Autodesk Fusion 360 part; units mm, degrees
(part 6 of 7)
  spline S7 degree 5 poles (-3.0907, -4.5495) (-3.0883, -4.5484) (-3.0835, -4.5462) (-3.0762, -4.5428) (-3.0666, -4.5384) (-3.0547, -4.5328) (-3.0428, -4.5271) (-3.0309, -4.5214) (-3.0191, -4.5157) (-3.0074, -4.5099) (-2.9957, -4.504) (-2.984, -4.4981) (-2.9724, -4.4922) (-2.9609, -4.4862) (-2.9494, -4.4802) (-2.9379, -4.4741) (-2.9265, -4.468) (-2.9152, -4.4618) (-2.9039, -4.4556) (-2.8926, -4.4494) (-2.8814, -4.443) (-2.8703, -4.4367) (-2.8592, -4.4303) (-2.8482, -4.4238) (-2.8372, -4.4173) (-2.8263, -4.4108) (-2.8154, -4.4042) (-2.8046, -4.3976) (-2.7939, -4.3909) (-2.7832, -4.3841) (-2.7726, -4.3773) (-2.762, -4.3705) (-2.7515, -4.3636) (-2.741, -4.3567) (-2.7306, -4.3497) (-2.7203, -4.3427) (-2.71, -4.3356) (-2.6998, -4.3285) (-2.6897, -4.3213) (-2.6796, -4.3141) (-2.6696, -4.3068) (-2.6597, -4.2995) (-2.6498, -4.2921) (-2.64, -4.2847) (-2.6303, -4.2772) (-2.6206, -4.2697) (-2.611, -4.2621) (-2.6015, -4.2544) (-2.5921, -4.2467) (-2.5827, -4.239) (-2.5734, -4.2312) (-2.5642, -4.2233) (-2.5551, -4.2154) (-2.5461, -4.2074) (-2.5371, -4.1994) (-2.5282, -4.1913) (-2.5195, -4.1831) (-2.5107, -4.1749) (-2.5021, -4.1667) (-2.4936, -4.1583) (-2.4852, -4.1499) (-2.4769, -4.1415) (-2.4687, -4.1329) (-2.4607, -4.1242) (-2.4528, -4.1155) (-2.445, -4.1067) (-2.4373, -4.0978) (-2.4297, -4.0889) (-2.4221, -4.08) (-2.4148, -4.0709) (-2.4077, -4.0616) (-2.4024, -4.054) (-2.3986, -4.0482) (-2.3962, -4.0442) (-2.395, -4.0422) knots -1 -1 -1 -1 -1 -1 -0.98571429 -0.97142857 -0.95714286 -0.94285714 -0.92857143 -0.91428571 -0.9 -0.88571429 -0.87142857 -0.85714286 -0.84285714 -0.82857143 -0.81428571 -0.8 -0.78571429 -0.77142857 -0.75714286 -0.74285714 -0.72857143 -0.71428571 -0.7 -0.68571429 -0.67142857 -0.65714286 -0.64285714 -0.62857143 -0.61428571 -0.6 -0.58571429 -0.57142857 -0.55714286 -0.54285714 -0.52857143 -0.51428571 -0.5 -0.48571429 -0.47142857 -0.45714286 -0.44285714 -0.42857143 -0.41428571 -0.4 -0.38571429 -0.37142857 -0.35714286 -0.34285714 -0.32857143 -0.31428571 -0.3 -0.28571429 -0.27142857 -0.25714286 -0.24285714 -0.22857143 -0.21428571 -0.2 -0.18571429 -0.17142857 -0.15714286 -0.14285714 -0.12857143 -0.11428571 -0.1 -0.08571429 -0.07142857 -0.05714286 -0.04285714 -0.02857143 -0.01428571 0 0 0 0 0 0
  line L7 (-2.395, -4.0422) -> (-2.2666, -3.8269)
  arc A15 (-2.1317, -3.791) -> (-2.2666, -3.8269) centre (-2.1807, -3.8781) ccw
  arc A16 (-2.1317, -3.791) -> (-1.814, -3.9529) centre (0, 0) ccw
  arc A17 (-1.7637, -4.0832) -> (-1.814, -3.9529) centre (-1.8557, -4.0437) ccw
  line L8 (-1.7637, -4.0832) -> (-1.8625, -4.3135)
  spline S8 degree 5 poles (-1.8625, -4.3135) (-1.8634, -4.3157) (-1.8652, -4.32) (-1.8677, -4.3265) (-1.8707, -4.3353) (-1.8741, -4.3464) (-1.8771, -4.3577) (-1.8799, -4.3691) (-1.8826, -4.3805) (-1.8852, -4.3919) (-1.8877, -4.4034) (-1.8902, -4.4149) (-1.8925, -4.4265) (-1.8946, -4.4381) (-1.8966, -4.4498) (-1.8985, -4.4616) (-1.9002, -4.4734) (-1.9018, -4.4852) (-1.9033, -4.4971) (-1.9047, -4.509) (-1.9061, -4.5209) (-1.9073, -4.5329) (-1.9085, -4.5449) (-1.9095, -4.5569) (-1.9105, -4.569) (-1.9113, -4.5811) (-1.9121, -4.5932) (-1.9128, -4.6054) (-1.9134, -4.6176) (-1.9139, -4.6298) (-1.9143, -4.642) (-1.9146, -4.6543) (-1.9149, -4.6666) (-1.915, -4.6789) (-1.9151, -4.6913) (-1.9151, -4.7036) (-1.9151, -4.716) (-1.9149, -4.7284) (-1.9147, -4.7409) (-1.9144, -4.7533) (-1.914, -4.7658) (-1.9135, -4.7783) (-1.913, -4.7909) (-1.9124, -4.8034) (-1.9117, -4.816) (-1.9109, -4.8286) (-1.9101, -4.8412) (-1.9092, -4.8538) (-1.9082, -4.8664) (-1.9072, -4.8791) (-1.906, -4.8918) (-1.9048, -4.9045) (-1.9036, -4.9172) (-1.9022, -4.9299) (-1.9008, -4.9427) (-1.8994, -4.9554) (-1.8978, -4.9682) (-1.8962, -4.981) (-1.8945, -4.9938) (-1.8928, -5.0066) (-1.891, -5.0195) (-1.8891, -5.0323) (-1.8871, -5.0452) (-1.8851, -5.0581) (-1.883, -5.071) (-1.8809, -5.0839) (-1.8787, -5.0968) (-1.8764, -5.1097) (-1.874, -5.1227) (-1.8716, -5.1356) (-1.8691, -5.1486) (-1.8671, -5.1589) (-1.8655, -5.1667) (-1.8645, -5.1719) (-1.8639, -5.1745) knots 0 0 0 0 0 0 0.01428571 0.02857143 0.04285714 0.05714286 0.07142857 0.08571429 0.1 0.11428571 0.12857143 0.14285714 0.15714286 0.17142857 0.18571429 0.2 0.21428571 0.22857143 0.24285714 0.25714286 0.27142857 0.28571429 0.3 0.31428571 0.32857143 0.34285714 0.35714286 0.37142857 0.38571429 0.4 0.41428571 0.42857143 0.44285714 0.45714286 0.47142857 0.48571429 0.5 0.51428571 0.52857143 0.54285714 0.55714286 0.57142857 0.58571429 0.6 0.61428571 0.62857143 0.64285714 0.65714286 0.67142857 0.68571429 0.7 0.71428571 0.72857143 0.74285714 0.75714286 0.77142857 0.78571429 0.8 0.81428571 0.82857143 0.84285714 0.85714286 0.87142857 0.88571429 0.9 0.91428571 0.92857143 0.94285714 0.95714286 0.97142857 0.98571429 1 1 1 1 1 1
  arc A18 (-1.8639, -5.1745) -> (-1.5336, -5.2819) centre (0, 0) ccw
  spline S9 degree 5 poles (-1.5336, -5.2819) (-1.5316, -5.2801) (-1.5277, -5.2765) (-1.5219, -5.2711) (-1.5141, -5.2639) (-1.5045, -5.2549) (-1.4949, -5.2458) (-1.4854, -5.2367) (-1.476, -5.2276) (-1.4666, -5.2185) (-1.4572, -5.2093) (-1.448, -5.2001) (-1.4388, -5.1909) (-1.4296, -5.1816) (-1.4206, -5.1723) (-1.4115, -5.163) (-1.4026, -5.1537) (-1.3937, -5.1443) (-1.3849, -5.1349) (-1.3761, -5.1255) (-1.3674, -5.116) (-1.3588, -5.1065) (-1.3502, -5.097) (-1.3417, -5.0875) (-1.3333, -5.0779) (-1.3249, -5.0683) (-1.3167, -5.0587) (-1.3084, -5.049) (-1.3003, -5.0393) (-1.2922, -5.0296) (-1.2842, -5.0199) (-1.2762, -5.0101) (-1.2684, -5.0003) (-1.2606, -4.9905) (-1.2528, -4.9806) (-1.2452, -4.9708) (-1.2376, -4.9609) (-1.2301, -4.9509) (-1.2227, -4.941) (-1.2154, -4.931) (-1.2081, -4.921) (-1.2009, -4.9109) (-1.1938, -4.9009) (-1.1868, -4.8908) (-1.1798, -4.8807) (-1.173, -4.8705) (-1.1662, -4.8603) (-1.1595, -4.8501) (-1.1529, -4.8399) (-1.1464, -4.8296) (-1.14, -4.8193) (-1.1336, -4.809) (-1.1274, -4.7987) (-1.1213, -4.7883) (-1.1153, -4.7779) (-1.1093, -4.7674) (-1.1035, -4.7569) (-1.0977, -4.7465) (-1.0921, -4.7359) (-1.0865, -4.7254) (-1.0811, -4.7148) (-1.0759, -4.7042) (-1.0708, -4.6935) (-1.0659, -4.6828) (-1.061, -4.672) (-1.0564, -4.6612) (-1.0517, -4.6504) (-1.0472, -4.6396) (-1.0428, -4.6288) (-1.0386, -4.6179) (-1.0348, -4.6069) (-1.032, -4.598) (-1.0302, -4.5913) (-1.0291, -4.5868) (-1.0286, -4.5845) knots -1 -1 -1 -1 -1 -1 -0.98571429 -0.97142857 -0.95714286 -0.94285714 -0.92857143 -0.91428571 -0.9 -0.88571429 -0.87142857 -0.85714286 -0.84285714 -0.82857143 -0.81428571 -0.8 -0.78571429 -0.77142857 -0.75714286 -0.74285714 -0.72857143 -0.71428571 -0.7 -0.68571429 -0.67142857 -0.65714286 -0.64285714 -0.62857143 -0.61428571 -0.6 -0.58571429 -0.57142857 -0.55714286 -0.54285714 -0.52857143 -0.51428571 -0.5 -0.48571429 -0.47142857 -0.45714286 -0.44285714 -0.42857143 -0.41428571 -0.4 -0.38571429 -0.37142857 -0.35714286 -0.34285714 -0.32857143 -0.31428571 -0.3 -0.28571429 -0.27142857 -0.25714286 -0.24285714 -0.22857143 -0.21428571 -0.2 -0.18571429 -0.17142857 -0.15714286 -0.14285714 -0.12857143 -0.11428571 -0.1 -0.08571429 -0.07142857 -0.05714286 -0.04285714 -0.02857143 -0.01428571 0 0 0 0 0 0
  line L9 (-1.0286, -4.5845) -> (-0.9731, -4.34)
  arc A19 (-0.8559, -4.2641) -> (-0.9731, -4.34) centre (-0.8756, -4.3622) ccw
  arc A20 (-0.8559, -4.2641) -> (-0.5037, -4.3199) centre (0, 0) ccw
  arc A21 (-0.4157, -4.4283) -> (-0.5037, -4.3199) centre (-0.5152, -4.4193) ccw
  line L10 (-0.4157, -4.4283) -> (-0.4384, -4.678)
  spline S10 degree 5 poles (-0.4384, -4.678) (-0.4386, -4.6803) (-0.439, -4.6849) (-0.4393, -4.6919) (-0.4395, -4.7012) (-0.4392, -4.7128) (-0.4386, -4.7245) (-0.4378, -4.7361) (-0.4368, -4.7478) (-0.4357, -4.7595) (-0.4346, -4.7712) (-0.4334, -4.7829) (-0.432, -4.7947) (-0.4304, -4.8064) (-0.4287, -4.8181) (-0.4269, -4.8299) (-0.4248, -4.8416) (-0.4227, -4.8534) (-0.4205, -4.8651) (-0.4182, -4.8769) (-0.4158, -4.8886) (-0.4133, -4.9004) (-0.4106, -4.9122) (-0.4079, -4.9239) (-0.4051, -4.9357) (-0.4022, -4.9475) (-0.3991, -4.9593) (-0.396, -4.971) (-0.3928, -4.9828) (-0.3895, -4.9946) (-0.3861, -5.0064) (-0.3826, -5.0181) (-0.3791, -5.0299) (-0.3754, -5.0417) (-0.3717, -5.0535) (-0.3679, -5.0652) (-0.364, -5.077) (-0.36, -5.0888) (-0.3559, -5.1005) (-0.3518, -5.1123) (-0.3476, -5.124) (-0.3433, -5.1358) (-0.3389, -5.1475) (-0.3344, -5.1593) (-0.3299, -5.171) (-0.3253, -5.1828) (-0.3206, -5.1945) (-0.3158, -5.2062) (-0.311, -5.2179) (-0.3061, -5.2297) (-0.3011, -5.2414) (-0.296, -5.2531) (-0.2909, -5.2648) (-0.2857, -5.2765) (-0.2804, -5.2882) (-0.2751, -5.2998) (-0.2697, -5.3115) (-0.2642, -5.3232) (-0.2586, -5.3348) (-0.253, -5.3465) (-0.2473, -5.3581) (-0.2415, -5.3698) (-0.2357, -5.3814) (-0.2298, -5.393) (-0.2238, -5.4047) (-0.2178, -5.4163) (-0.2117, -5.4279) (-0.2055, -5.4395) (-0.1993, -5.451) (-0.193, -5.4626) (-0.1866, -5.4742) (-0.1815, -5.4834) (-0.1776, -5.4903) (-0.175, -5.4949) (-0.1737, -5.4973) knots 0 0 0 0 0 0 0.01428571 0.02857143 0.04285714 0.05714286 0.07142857 0.08571429 0.1 0.11428571 0.12857143 0.14285714 0.15714286 0.17142857 0.18571429 0.2 0.21428571 0.22857143 0.24285714 0.25714286 0.27142857 0.28571429 0.3 0.31428571 0.32857143 0.34285714 0.35714286 0.37142857 0.38571429 0.4 0.41428571 0.42857143 0.44285714 0.45714286 0.47142857 0.48571429 0.5 0.51428571 0.52857143 0.54285714 0.55714286 0.57142857 0.58571429 0.6 0.61428571 0.62857143 0.64285714 0.65714286 0.67142857 0.68571429 0.7 0.71428571 0.72857143 0.74285714 0.75714286 0.77142857 0.78571429 0.8 0.81428571 0.82857143 0.84285714 0.85714286 0.87142857 0.88571429 0.9 0.91428571 0.92857143 0.94285714 0.95714286 0.97142857 0.98571429 1 1 1 1 1 1
  arc A22 (-0.1737, -5.4973) -> (0.1737, -5.4973) centre (0, 0) ccw
  spline S11 degree 5 poles (0.1737, -5.4973) (0.175, -5.4949) (0.1776, -5.4903) (0.1815, -5.4834) (0.1866, -5.4742) (0.193, -5.4626) (0.1993, -5.451) (0.2055, -5.4395) (0.2117, -5.4279) (0.2178, -5.4163) (0.2238, -5.4047) (0.2298, -5.393) (0.2357, -5.3814) (0.2415, -5.3698) (0.2473, -5.3581) (0.253, -5.3465) (0.2586, -5.3348) (0.2642, -5.3232) (0.2697, -5.3115) (0.2751, -5.2998) (0.2804, -5.2882) (0.2857, -5.2765) (0.2909, -5.2648) (0.296, -5.2531) (0.3011, -5.2414) (0.3061, -5.2297) (0.311, -5.2179) (0.3158, -5.2062) (0.3206, -5.1945) (0.3253, -5.1828) (0.3299, -5.171) (0.3344, -5.1593) (0.3389, -5.1475) (0.3433, -5.1358) (0.3476, -5.124) (0.3518, -5.1123) (0.3559, -5.1005) (0.36, -5.0888) (0.364, -5.077) (0.3679, -5.0652) (0.3717, -5.0535) (0.3754, -5.0417) (0.3791, -5.0299) (0.3826, -5.0181) (0.3861, -5.0064) (0.3895, -4.9946) (0.3928, -4.9828) (0.396, -4.971) (0.3991, -4.9593) (0.4022, -4.9475) (0.4051, -4.9357) (0.4079, -4.9239) (0.4106, -4.9122) (0.4133, -4.9004) (0.4158, -4.8886) (0.4182, -4.8769) (0.4205, -4.8651) (0.4227, -4.8534) (0.4248, -4.8416) (0.4269, -4.8299) (0.4287, -4.8181) (0.4304, -4.8064) (0.432, -4.7947) (0.4334, -4.7829) (0.4346, -4.7712) (0.4357, -4.7595) (0.4368, -4.7478) (0.4378, -4.7361) (0.4386, -4.7245) (0.4392, -4.7128) (0.4395, -4.7012) (0.4393, -4.6919) (0.439, -4.6849) (0.4386, -4.6803) (0.4384, -4.678) knots -1 -1 -1 -1 -1 -1 -0.98571429 -0.97142857 -0.95714286 -0.94285714 -0.92857143 -0.91428571 -0.9 -0.88571429 -0.87142857 -0.85714286 -0.84285714 -0.82857143 -0.81428571 -0.8 -0.78571429 -0.77142857 -0.75714286 -0.74285714 -0.72857143 -0.71428571 -0.7 -0.68571429 -0.67142857 -0.65714286 -0.64285714 -0.62857143 -0.61428571 -0.6 -0.58571429 -0.57142857 -0.55714286 -0.54285714 -0.52857143 -0.51428571 -0.5 -0.48571429 -0.47142857 -0.45714286 -0.44285714 -0.42857143 -0.41428571 -0.4 -0.38571429 -0.37142857 -0.35714286 -0.34285714 -0.32857143 -0.31428571 -0.3 -0.28571429 -0.27142857 -0.25714286 -0.24285714 -0.22857143 -0.21428571 -0.2 -0.18571429 -0.17142857 -0.15714286 -0.14285714 -0.12857143 -0.11428571 -0.1 -0.08571429 -0.07142857 -0.05714286 -0.04285714 -0.02857143 -0.01428571 0 0 0 0 0 0
  line L11 (0.4384, -4.678) -> (0.4157, -4.4283)
  arc A23 (0.5037, -4.3199) -> (0.4157, -4.4283) centre (0.5152, -4.4193) ccw
  arc A24 (0.5037, -4.3199) -> (0.8559, -4.2641) centre (0, 0) ccw
  arc A25 (0.9731, -4.34) -> (0.8559, -4.2641) centre (0.8756, -4.3622) ccw
  line L12 (0.9731, -4.34) -> (1.0286, -4.5845)
  spline S12 degree 5 poles (1.0286, -4.5845) (1.0291, -4.5868) (1.0302, -4.5913) (1.032, -4.598) (1.0348, -4.6069) (1.0386, -4.6179) (1.0428, -4.6288) (1.0472, -4.6396) (1.0517, -4.6504) (1.0564, -4.6612) (1.061, -4.672) (1.0659, -4.6828) (1.0708, -4.6935) (1.0759, -4.7042) (1.0811, -4.7148) (1.0865, -4.7254) (1.0921, -4.7359) (1.0977, -4.7465) (1.1035, -4.7569) (1.1093, -4.7674) (1.1153, -4.7779) (1.1213, -4.7883) (1.1274, -4.7987) (1.1336, -4.809) (1.14, -4.8193) (1.1464, -4.8296) (1.1529, -4.8399) (1.1595, -4.8501) (1.1662, -4.8603) (1.173, -4.8705) (1.1798, -4.8807) (1.1868, -4.8908) (1.1938, -4.9009) (1.2009, -4.9109) (1.2081, -4.921) (1.2154, -4.931) (1.2227, -4.941) (1.2301, -4.9509) (1.2376, -4.9609) (1.2452, -4.9708) (1.2528, -4.9806) (1.2606, -4.9905) (1.2684, -5.0003) (1.2762, -5.0101) (1.2842, -5.0199) (1.2922, -5.0296) (1.3003, -5.0393) (1.3084, -5.049) (1.3167, -5.0587) (1.3249, -5.0683) (1.3333, -5.0779) (1.3417, -5.0875) (1.3502, -5.097) (1.3588, -5.1065) (1.3674, -5.116) (1.3761, -5.1255) (1.3849, -5.1349) (1.3937, -5.1443) (1.4026, -5.1537) (1.4115, -5.163) (1.4206, -5.1723) (1.4296, -5.1816) (1.4388, -5.1909) (1.448, -5.2001) (1.4572, -5.2093) (1.4666, -5.2185) (1.476, -5.2276) (1.4854, -5.2367) (1.4949, -5.2458) (1.5045, -5.2549) (1.5141, -5.2639) (1.5219, -5.2711) (1.5277, -5.2765) (1.5316, -5.2801) (1.5336, -5.2819) knots 0 0 0 0 0 0 0.01428571 0.02857143 0.04285714 0.05714286 0.07142857 0.08571429 0.1 0.11428571 0.12857143 0.14285714 0.15714286 0.17142857 0.18571429 0.2 0.21428571 0.22857143 0.24285714 0.25714286 0.27142857 0.28571429 0.3 0.31428571 0.32857143 0.34285714 0.35714286 0.37142857 0.38571429 0.4 0.41428571 0.42857143 0.44285714 0.45714286 0.47142857 0.48571429 0.5 0.51428571 0.52857143 0.54285714 0.55714286 0.57142857 0.58571429 0.6 0.61428571 0.62857143 0.64285714 0.65714286 0.67142857 0.68571429 0.7 0.71428571 0.72857143 0.74285714 0.75714286 0.77142857 0.78571429 0.8 0.81428571 0.82857143 0.84285714 0.85714286 0.87142857 0.88571429 0.9 0.91428571 0.92857143 0.94285714 0.95714286 0.97142857 0.98571429 1 1 1 1 1 1
  arc A26 (1.5336, -5.2819) -> (1.8639, -5.1745) centre (0, 0) ccw
  spline S13 degree 5 poles (1.8639, -5.1745) (1.8645, -5.1719) (1.8655, -5.1667) (1.8671, -5.1589) (1.8691, -5.1486) (1.8716, -5.1356) (1.874, -5.1227) (1.8764, -5.1097) (1.8787, -5.0968) (1.8809, -5.0839) (1.883, -5.071) (1.8851, -5.0581) (1.8871, -5.0452) (1.8891, -5.0323) (1.891, -5.0195) (1.8928, -5.0066) (1.8945, -4.9938) (1.8962, -4.981) (1.8978, -4.9682) (1.8994, -4.9554) (1.9008, -4.9427) (1.9022, -4.9299) (1.9036, -4.9172) (1.9048, -4.9045) (1.906, -4.8918) (1.9072, -4.8791) (1.9082, -4.8664) (1.9092, -4.8538) (1.9101, -4.8412) (1.9109, -4.8286) (1.9117, -4.816) (1.9124, -4.8034) (1.913, -4.7909) (1.9135, -4.7783) (1.914, -4.7658) (1.9144, -4.7533) (1.9147, -4.7409) (1.9149, -4.7284) (1.9151, -4.716) (1.9151, -4.7036) (1.9151, -4.6913) (1.915, -4.6789) (1.9149, -4.6666) (1.9146, -4.6543) (1.9143, -4.642) (1.9139, -4.6298) (1.9134, -4.6176) (1.9128, -4.6054) (1.9121, -4.5932) (1.9113, -4.5811) (1.9105, -4.569) (1.9095, -4.5569) (1.9085, -4.5449) (1.9073, -4.5329) (1.9061, -4.5209) (1.9047, -4.509) (1.9033, -4.4971) (1.9018, -4.4852) (1.9002, -4.4734) (1.8985, -4.4616) (1.8966, -4.4498) (1.8946, -4.4381) (1.8925, -4.4265) (1.8902, -4.4149) (1.8877, -4.4034) (1.8852, -4.3919) (1.8826, -4.3805) (1.8799, -4.3691) (1.8771, -4.3577) (1.8741, -4.3464) (1.8707, -4.3353) (1.8677, -4.3265) (1.8652, -4.32) (1.8634, -4.3157) (1.8625, -4.3135) knots -1 -1 -1 -1 -1 -1 -0.98571429 -0.97142857 -0.95714286 -0.94285714 -0.92857143 -0.91428571 -0.9 -0.88571429 -0.87142857 -0.85714286 -0.84285714 -0.82857143 -0.81428571 -0.8 -0.78571429 -0.77142857 -0.75714286 -0.74285714 -0.72857143 -0.71428571 -0.7 -0.68571429 -0.67142857 -0.65714286 -0.64285714 -0.62857143 -0.61428571 -0.6 -0.58571429 -0.57142857 -0.55714286 -0.54285714 -0.52857143 -0.51428571 -0.5 -0.48571429 -0.47142857 -0.45714286 -0.44285714 -0.42857143 -0.41428571 -0.4 -0.38571429 -0.37142857 -0.35714286 -0.34285714 -0.32857143 -0.31428571 -0.3 -0.28571429 -0.27142857 -0.25714286 -0.24285714 -0.22857143 -0.21428571 -0.2 -0.18571429 -0.17142857 -0.15714286 -0.14285714 -0.12857143 -0.11428571 -0.1 -0.08571429 -0.07142857 -0.05714286 -0.04285714 -0.02857143 -0.01428571 0 0 0 0 0 0
  line L13 (1.8625, -4.3135) -> (1.7637, -4.0832)
  arc A27 (1.814, -3.9529) -> (1.7637, -4.0832) centre (1.8557, -4.0437) ccw
  arc A28 (1.814, -3.9529) -> (2.1317, -3.791) centre (0, 0) ccw
  arc A29 (2.2666, -3.8269) -> (2.1317, -3.791) centre (2.1807, -3.8781) ccw
  line L14 (2.2666, -3.8269) -> (2.395, -4.0422)
  spline S14 degree 5 poles (2.395, -4.0422) (2.3962, -4.0442) (2.3986, -4.0482) (2.4024, -4.054) (2.4077, -4.0616) (2.4148, -4.0709) (2.4221, -4.08) (2.4297, -4.0889) (2.4373, -4.0978) (2.445, -4.1067) (2.4528, -4.1155) (2.4607, -4.1242) (2.4687, -4.1329) (2.4769, -4.1415) (2.4852, -4.1499) (2.4936, -4.1583) (2.5021, -4.1667) (2.5107, -4.1749) (2.5195, -4.1831) (2.5282, -4.1913) (2.5371, -4.1994) (2.5461, -4.2074) (2.5551, -4.2154) (2.5642, -4.2233) (2.5734, -4.2312) (2.5827, -4.239) (2.5921, -4.2467) (2.6015, -4.2544) (2.611, -4.2621) (2.6206, -4.2697) (2.6303, -4.2772) (2.64, -4.2847) (2.6498, -4.2921) (2.6597, -4.2995) (2.6696, -4.3068) (2.6796, -4.3141) (2.6897, -4.3213) (2.6998, -4.3285) (2.71, -4.3356) (2.7203, -4.3427) (2.7306, -4.3497) (2.741, -4.3567) (2.7515, -4.3636) (2.762, -4.3705) (2.7726, -4.3773) (2.7832, -4.3841) (2.7939, -4.3909) (2.8046, -4.3976) (2.8154, -4.4042) (2.8263, -4.4108) (2.8372, -4.4173) (2.8482, -4.4238) (2.8592, -4.4303) (2.8703, -4.4367) (2.8814, -4.443) (2.8926, -4.4494) (2.9039, -4.4556) (2.9152, -4.4618) (2.9265, -4.468) (2.9379, -4.4741) (2.9494, -4.4802) (2.9609, -4.4862) (2.9724, -4.4922) (2.984, -4.4981) (2.9957, -4.504) (3.0074, -4.5099) (3.0191, -4.5157) (3.0309, -4.5214) (3.0428, -4.5271) (3.0547, -4.5328) (3.0666, -4.5384) (3.0762, -4.5428) (3.0835, -4.5462) (3.0883, -4.5484) (3.0907, -4.5495) knots 0 0 0 0 0 0 0.01428571 0.02857143 0.04285714 0.05714286 0.07142857 0.08571429 0.1 0.11428571 0.12857143 0.14285714 0.15714286 0.17142857 0.18571429 0.2 0.21428571 0.22857143 0.24285714 0.25714286 0.27142857 0.28571429 0.3 0.31428571 0.32857143 0.34285714 0.35714286 0.37142857 0.38571429 0.4 0.41428571 0.42857143 0.44285714 0.45714286 0.47142857 0.48571429 0.5 0.51428571 0.52857143 0.54285714 0.55714286 0.57142857 0.58571429 0.6 0.61428571 0.62857143 0.64285714 0.65714286 0.67142857 0.68571429 0.7 0.71428571 0.72857143 0.74285714 0.75714286 0.77142857 0.78571429 0.8 0.81428571 0.82857143 0.84285714 0.85714286 0.87142857 0.88571429 0.9 0.91428571 0.92857143 0.94285714 0.95714286 0.97142857 0.98571429 1 1 1 1 1 1
  arc A30 (3.0907, -4.5495) -> (3.3717, -4.3453) centre (0, 0) ccw
  spline S15 degree 5 poles (3.3717, -4.3453) (3.3714, -4.3426) (3.3708, -4.3374) (3.3699, -4.3295) (3.3686, -4.319) (3.367, -4.3059) (3.3653, -4.2928) (3.3635, -4.2798) (3.3617, -4.2668) (3.3598, -4.2538) (3.3579, -4.2409) (3.3559, -4.228) (3.3538, -4.2151) (3.3517, -4.2023) (3.3495, -4.1895) (3.3473, -4.1767) (3.345, -4.164) (3.3426, -4.1513) (3.3402, -4.1386) (3.3377, -4.126) (3.3352, -4.1134) (3.3326, -4.1008) (3.3299, -4.0883) (3.3272, -4.0758) (3.3244, -4.0634) (3.3215, -4.051) (3.3186, -4.0386) (3.3157, -4.0263) (3.3126, -4.014) (3.3095, -4.0017) (3.3063, -3.9895) (3.3031, -3.9774) (3.2998, -3.9652) (3.2964, -3.9532) (3.293, -3.9411) (3.2895, -3.9291) (3.286, -3.9172) (3.2823, -3.9053) (3.2787, -3.8934) (3.2749, -3.8816) (3.2711, -3.8698) (3.2672, -3.8581) (3.2632, -3.8465) (3.2592, -3.8348) (3.255, -3.8233) (3.2509, -3.8118) (3.2466, -3.8003) (3.2423, -3.7889) (3.2379, -3.7775) (3.2334, -3.7662) (3.2289, -3.755) (3.2242, -3.7438) (3.2195, -3.7327) (3.2147, -3.7216) (3.2098, -3.7106) (3.2049, -3.6997) (3.1998, -3.6888) (3.1947, -3.678) (3.1895, -3.6672) (3.1843, -3.6565) (3.1789, -3.6459) (3.1734, -3.6354) (3.1677, -3.625) (3.1619, -3.6148) (3.1561, -3.6045) (3.1501, -3.5944) (3.1441, -3.5843) (3.138, -3.5743) (3.1318, -3.5644) (3.1254, -3.5546) (3.1188, -3.545) (3.1132, -3.5376) (3.1089, -3.5321) (3.1058, -3.5286) (3.1043, -3.5269) knots -1 -1 -1 -1 -1 -1 -0.98571429 -0.97142857 -0.95714286 -0.94285714 -0.92857143 -0.91428571 -0.9 -0.88571429 -0.87142857 -0.85714286 -0.84285714 -0.82857143 -0.81428571 -0.8 -0.78571429 -0.77142857 -0.75714286 -0.74285714 -0.72857143 -0.71428571 -0.7 -0.68571429 -0.67142857 -0.65714286 -0.64285714 -0.62857143 -0.61428571 -0.6 -0.58571429 -0.57142857 -0.55714286 -0.54285714 -0.52857143 -0.51428571 -0.5 -0.48571429 -0.47142857 -0.45714286 -0.44285714 -0.42857143 -0.41428571 -0.4 -0.38571429 -0.37142857 -0.35714286 -0.34285714 -0.32857143 -0.31428571 -0.3 -0.28571429 -0.27142857 -0.25714286 -0.24285714 -0.22857143 -0.21428571 -0.2 -0.18571429 -0.17142857 -0.15714286 -0.14285714 -0.12857143 -0.11428571 -0.1 -0.08571429 -0.07142857 -0.05714286 -0.04285714 -0.02857143 -0.01428571 0 0 0 0 0 0
  line L15 (3.1043, -3.5269) -> (2.9392, -3.3383)
  arc A31 (2.9467, -3.1989) -> (2.9392, -3.3383) centre (3.0144, -3.2724) ccw
  arc A32 (2.9467, -3.1989) -> (3.1989, -2.9467) centre (0, 0) ccw
  arc A33 (3.3383, -2.9392) -> (3.1989, -2.9467) centre (3.2724, -3.0144) ccw
  line L16 (3.3383, -2.9392) -> (3.5269, -3.1043)
  spline S16 degree 5 poles (3.5269, -3.1043) (3.5286, -3.1058) (3.5321, -3.1089) (3.5376, -3.1132) (3.545, -3.1188) (3.5546, -3.1254) (3.5644, -3.1318) (3.5743, -3.138) (3.5843, -3.1441) (3.5944, -3.1501) (3.6045, -3.1561) (3.6148, -3.1619) (3.625, -3.1677) (3.6354, -3.1734) (3.6459, -3.1789) (3.6565, -3.1843) (3.6672, -3.1895) (3.678, -3.1947) (3.6888, -3.1998) (3.6997, -3.2049) (3.7106, -3.2098) (3.7216, -3.2147) (3.7327, -3.2195) (3.7438, -3.2242) (3.755, -3.2289) (3.7662, -3.2334) (3.7775, -3.2379) (3.7889, -3.2423) (3.8003, -3.2466) (3.8118, -3.2509) (3.8233, -3.255) (3.8348, -3.2592) (3.8465, -3.2632) (3.8581, -3.2672) (3.8698, -3.2711) (3.8816, -3.2749) (3.8934, -3.2787) (3.9053, -3.2823) (3.9172, -3.286) (3.9291, -3.2895) (3.9411, -3.293) (3.9532, -3.2964) (3.9652, -3.2998) (3.9774, -3.3031) (3.9895, -3.3063) (4.0017, -3.3095) (4.014, -3.3126) (4.0263, -3.3157) (4.0386, -3.3186) (4.051, -3.3215) (4.0634, -3.3244) (4.0758, -3.3272) (4.0883, -3.3299) (4.1008, -3.3326) (4.1134, -3.3352) (4.126, -3.3377) (4.1386, -3.3402) (4.1513, -3.3426) (4.164, -3.345) (4.1767, -3.3473) (4.1895, -3.3495) (4.2023, -3.3517) (4.2151, -3.3538) (4.228, -3.3559) (4.2409, -3.3579) (4.2538, -3.3598) (4.2668, -3.3617) (4.2798, -3.3635) (4.2928, -3.3653) (4.3059, -3.367) (4.319, -3.3686) (4.3295, -3.3699) (4.3374, -3.3708) (4.3426, -3.3714) (4.3453, -3.3717) knots 0 0 0 0 0 0 0.01428571 0.02857143 0.04285714 0.05714286 0.07142857 0.08571429 0.1 0.11428571 0.12857143 0.14285714 0.15714286 0.17142857 0.18571429 0.2 0.21428571 0.22857143 0.24285714 0.25714286 0.27142857 0.28571429 0.3 0.31428571 0.32857143 0.34285714 0.35714286 0.37142857 0.38571429 0.4 0.41428571 0.42857143 0.44285714 0.45714286 0.47142857 0.48571429 0.5 0.51428571 0.52857143 0.54285714 0.55714286 0.57142857 0.58571429 0.6 0.61428571 0.62857143 0.64285714 0.65714286 0.67142857 0.68571429 0.7 0.71428571 0.72857143 0.74285714 0.75714286 0.77142857 0.78571429 0.8 0.81428571 0.82857143 0.84285714 0.85714286 0.87142857 0.88571429 0.9 0.91428571 0.92857143 0.94285714 0.95714286 0.97142857 0.98571429 1 1 1 1 1 1
  arc A34 (4.3453, -3.3717) -> (4.5495, -3.0907) centre (0, 0) ccw
  spline S17 degree 5 poles (4.5495, -3.0907) (4.5484, -3.0883) (4.5462, -3.0835) (4.5428, -3.0762) (4.5384, -3.0666) (4.5328, -3.0547) (4.5271, -3.0428) (4.5214, -3.0309) (4.5157, -3.0191) (4.5099, -3.0074) (4.504, -2.9957) (4.4981, -2.984) (4.4922, -2.9724) (4.4862, -2.9609) (4.4802, -2.9494) (4.4741, -2.9379) (4.468, -2.9265) (4.4618, -2.9152) (4.4556, -2.9039) (4.4494, -2.8926) (4.443, -2.8814) (4.4367, -2.8703) (4.4303, -2.8592) (4.4238, -2.8482) (4.4173, -2.8372) (4.4108, -2.8263) (4.4042, -2.8154) (4.3976, -2.8046) (4.3909, -2.7939) (4.3841, -2.7832) (4.3773, -2.7726) (4.3705, -2.762) (4.3636, -2.7515) (4.3567, -2.741) (4.3497, -2.7306) (4.3427, -2.7203) (4.3356, -2.71) (4.3285, -2.6998) (4.3213, -2.6897) (4.3141, -2.6796) (4.3068, -2.6696) (4.2995, -2.6597) (4.2921, -2.6498) (4.2847, -2.64) (4.2772, -2.6303) (4.2697, -2.6206) (4.2621, -2.611) (4.2544, -2.6015) (4.2467, -2.5921) (4.239, -2.5827) (4.2312, -2.5734) (4.2233, -2.5642) (4.2154, -2.5551) (4.2074, -2.5461) (4.1994, -2.5371) (4.1913, -2.5282) (4.1831, -2.5195) (4.1749, -2.5107) (4.1667, -2.5021) (4.1583, -2.4936) (4.1499, -2.4852) (4.1415, -2.4769) (4.1329, -2.4687) (4.1242, -2.4607) (4.1155, -2.4528) (4.1067, -2.445) (4.0978, -2.4373) (4.0889, -2.4297) (4.08, -2.4221) (4.0709, -2.4148) (4.0616, -2.4077) (4.054, -2.4024) (4.0482, -2.3986) (4.0442, -2.3962) (4.0422, -2.395) knots -1 -1 -1 -1 -1 -1 -0.98571429 -0.97142857 -0.95714286 -0.94285714 -0.92857143 -0.91428571 -0.9 -0.88571429 -0.87142857 -0.85714286 -0.84285714 -0.82857143 -0.81428571 -0.8 -0.78571429 -0.77142857 -0.75714286 -0.74285714 -0.72857143 -0.71428571 -0.7 -0.68571429 -0.67142857 -0.65714286 -0.64285714 -0.62857143 -0.61428571 -0.6 -0.58571429 -0.57142857 -0.55714286 -0.54285714 -0.52857143 -0.51428571 -0.5 -0.48571429 -0.47142857 -0.45714286 -0.44285714 -0.42857143 -0.41428571 -0.4 -0.38571429 -0.37142857 -0.35714286 -0.34285714 -0.32857143 -0.31428571 -0.3 -0.28571429 -0.27142857 -0.25714286 -0.24285714 -0.22857143 -0.21428571 -0.2 -0.18571429 -0.17142857 -0.15714286 -0.14285714 -0.12857143 -0.11428571 -0.1 -0.08571429 -0.07142857 -0.05714286 -0.04285714 -0.02857143 -0.01428571 0 0 0 0 0 0
  line L17 (4.0422, -2.395) -> (3.8269, -2.2666)
  arc A35 (3.791, -2.1317) -> (3.8269, -2.2666) centre (3.8781, -2.1807) ccw
  arc A36 (3.791, -2.1317) -> (3.9529, -1.814) centre (0, 0) ccw
  arc A37 (4.0832, -1.7637) -> (3.9529, -1.814) centre (4.0437, -1.8557) ccw
  line L18 (4.0832, -1.7637) -> (4.3135, -1.8625)
  spline S18 degree 5 poles (4.3135, -1.8625) (4.3157, -1.8634) (4.32, -1.8652) (4.3265, -1.8677) (4.3353, -1.8707) (4.3464, -1.8741) (4.3577, -1.8771) (4.3691, -1.8799) (4.3805, -1.8826) (4.3919, -1.8852) (4.4034, -1.8877) (4.4149, -1.8902) (4.4265, -1.8925) (4.4381, -1.8946) (4.4498, -1.8966) (4.4616, -1.8985) (4.4734, -1.9002) (4.4852, -1.9018) (4.4971, -1.9033) (4.509, -1.9047) (4.5209, -1.9061) (4.5329, -1.9073) (4.5449, -1.9085) (4.5569, -1.9095) (4.569, -1.9105) (4.5811, -1.9113) (4.5932, -1.9121) (4.6054, -1.9128) (4.6176, -1.9134) (4.6298, -1.9139) (4.642, -1.9143) (4.6543, -1.9146) (4.6666, -1.9149) (4.6789, -1.915) (4.6913, -1.9151) (4.7036, -1.9151) (4.716, -1.9151) (4.7284, -1.9149) (4.7409, -1.9147) (4.7533, -1.9144) (4.7658, -1.914) (4.7783, -1.9135) (4.7909, -1.913) (4.8034, -1.9124) (4.816, -1.9117) (4.8286, -1.9109) (4.8412, -1.9101) (4.8538, -1.9092) (4.8664, -1.9082) (4.8791, -1.9072) (4.8918, -1.906) (4.9045, -1.9048) (4.9172, -1.9036) (4.9299, -1.9022) (4.9427, -1.9008) (4.9554, -1.8994) (4.9682, -1.8978) (4.981, -1.8962) (4.9938, -1.8945) (5.0066, -1.8928) (5.0195, -1.891) (5.0323, -1.8891) (5.0452, -1.8871) (5.0581, -1.8851) (5.071, -1.883) (5.0839, -1.8809) (5.0968, -1.8787) (5.1097, -1.8764) (5.1227, -1.874) (5.1356, -1.8716) (5.1486, -1.8691) (5.1589, -1.8671) (5.1667, -1.8655) (5.1719, -1.8645) (5.1745, -1.8639) knots 0 0 0 0 0 0 0.01428571 0.02857143 0.04285714 0.05714286 0.07142857 0.08571429 0.1 0.11428571 0.12857143 0.14285714 0.15714286 0.17142857 0.18571429 0.2 0.21428571 0.22857143 0.24285714 0.25714286 0.27142857 0.28571429 0.3 0.31428571 0.32857143 0.34285714 0.35714286 0.37142857 0.38571429 0.4 0.41428571 0.42857143 0.44285714 0.45714286 0.47142857 0.48571429 0.5 0.51428571 0.52857143 0.54285714 0.55714286 0.57142857 0.58571429 0.6 0.61428571 0.62857143 0.64285714 0.65714286 0.67142857 0.68571429 0.7 0.71428571 0.72857143 0.74285714 0.75714286 0.77142857 0.78571429 0.8 0.81428571 0.82857143 0.84285714 0.85714286 0.87142857 0.88571429 0.9 0.91428571 0.92857143 0.94285714 0.95714286 0.97142857 0.98571429 1 1 1 1 1 1
  arc A38 (5.1745, -1.8639) -> (5.2819, -1.5336) centre (0, 0) ccw
  spline S19 degree 5 poles (5.2819, -1.5336) (5.2801, -1.5316) (5.2765, -1.5277) (5.2711, -1.5219) (5.2639, -1.5141) (5.2549, -1.5045) (5.2458, -1.4949) (5.2367, -1.4854) (5.2276, -1.476) (5.2185, -1.4666) (5.2093, -1.4572) (5.2001, -1.448) (5.1909, -1.4388) (5.1816, -1.4296) (5.1723, -1.4206) (5.163, -1.4115) (5.1537, -1.4026) (5.1443, -1.3937) (5.1349, -1.3849) (5.1255, -1.3761) (5.116, -1.3674) (5.1065, -1.3588) (5.097, -1.3502) (5.0875, -1.3417) (5.0779, -1.3333) (5.0683, -1.3249) (5.0587, -1.3167) (5.049, -1.3084) (5.0393, -1.3003) (5.0296, -1.2922) (5.0199, -1.2842) (5.0101, -1.2762) (5.0003, -1.2684) (4.9905, -1.2606) (4.9806, -1.2528) (4.9708, -1.2452) (4.9609, -1.2376) (4.9509, -1.2301) (4.941, -1.2227) (4.931, -1.2154) (4.921, -1.2081) (4.9109, -1.2009) (4.9009, -1.1938) (4.8908, -1.1868) (4.8807, -1.1798) (4.8705, -1.173) (4.8603, -1.1662) (4.8501, -1.1595) (4.8399, -1.1529) (4.8296, -1.1464) (4.8193, -1.14) (4.809, -1.1336) (4.7987, -1.1274) (4.7883, -1.1213) (4.7779, -1.1153) (4.7674, -1.1093) (4.7569, -1.1035) (4.7465, -1.0977) (4.7359, -1.0921) (4.7254, -1.0865) (4.7148, -1.0811) (4.7042, -1.0759) (4.6935, -1.0708) (4.6828, -1.0659) (4.672, -1.061) (4.6612, -1.0564) (4.6504, -1.0517) (4.6396, -1.0472) (4.6288, -1.0428) (4.6179, -1.0386) (4.6069, -1.0348) (4.598, -1.032) (4.5913, -1.0302) (4.5868, -1.0291) (4.5845, -1.0286) knots -1 -1 -1 -1 -1 -1 -0.98571429 -0.97142857 -0.95714286 -0.94285714 -0.92857143 -0.91428571 -0.9 -0.88571429 -0.87142857 -0.85714286 -0.84285714 -0.82857143 -0.81428571 -0.8 -0.78571429 -0.77142857 -0.75714286 -0.74285714 -0.72857143 -0.71428571 -0.7 -0.68571429 -0.67142857 -0.65714286 -0.64285714 -0.62857143 -0.61428571 -0.6 -0.58571429 -0.57142857 -0.55714286 -0.54285714 -0.52857143 -0.51428571 -0.5 -0.48571429 -0.47142857 -0.45714286 -0.44285714 -0.42857143 -0.41428571 -0.4 -0.38571429 -0.37142857 -0.35714286 -0.34285714 -0.32857143 -0.31428571 -0.3 -0.28571429 -0.27142857 -0.25714286 -0.24285714 -0.22857143 -0.21428571 -0.2 -0.18571429 -0.17142857 -0.15714286 -0.14285714 -0.12857143 -0.11428571 -0.1 -0.08571429 -0.07142857 -0.05714286 -0.04285714 -0.02857143 -0.01428571 0 0 0 0 0 0
  line L19 (4.5845, -1.0286) -> (4.34, -0.9731)
  arc A39 (4.2641, -0.8559) -> (4.34, -0.9731) centre (4.3622, -0.8756) ccw
  arc A40 (4.2641, -0.8559) -> (4.3199, -0.5037) centre (0, 0) ccw
  arc A41 (4.4283, -0.4157) -> (4.3199, -0.5037) centre (4.4193, -0.5152) ccw
  line L20 (4.4283, -0.4157) -> (4.678, -0.4384)
  spline S20 degree 5 poles (4.678, -0.4384) (4.6803, -0.4386) (4.6849, -0.439) (4.6919, -0.4393) (4.7012, -0.4395) (4.7128, -0.4392) (4.7245, -0.4386) (4.7361, -0.4378) (4.7478, -0.4368) (4.7595, -0.4357) (4.7712, -0.4346) (4.7829, -0.4334) (4.7947, -0.432) (4.8064, -0.4304) (4.8181, -0.4287) (4.8299, -0.4269) (4.8416, -0.4248) (4.8534, -0.4227) (4.8651, -0.4205) (4.8769, -0.4182) (4.8886, -0.4158) (4.9004, -0.4133) (4.9122, -0.4106) (4.9239, -0.4079) (4.9357, -0.4051) (4.9475, -0.4022) (4.9593, -0.3991) (4.971, -0.396) (4.9828, -0.3928) (4.9946, -0.3895) (5.0064, -0.3861) (5.0181, -0.3826) (5.0299, -0.3791) (5.0417, -0.3754) (5.0535, -0.3717) (5.0652, -0.3679) (5.077, -0.364) (5.0888, -0.36) (5.1005, -0.3559) (5.1123, -0.3518) (5.124, -0.3476) (5.1358, -0.3433) (5.1475, -0.3389) (5.1593, -0.3344) (5.171, -0.3299) (5.1828, -0.3253) (5.1945, -0.3206) (5.2062, -0.3158) (5.2179, -0.311) (5.2297, -0.3061) (5.2414, -0.3011) (5.2531, -0.296) (5.2648, -0.2909) (5.2765, -0.2857) (5.2882, -0.2804) (5.2998, -0.2751) (5.3115, -0.2697) (5.3232, -0.2642) (5.3348, -0.2586) (5.3465, -0.253) (5.3581, -0.2473) (5.3698, -0.2415) (5.3814, -0.2357) (5.393, -0.2298) (5.4047, -0.2238) (5.4163, -0.2178) (5.4279, -0.2117) (5.4395, -0.2055) (5.451, -0.1993) (5.4626, -0.193) (5.4742, -0.1866) (5.4834, -0.1815) (5.4903, -0.1776) (5.4949, -0.175) (5.4973, -0.1737) knots 0 0 0 0 0 0 0.01428571 0.02857143 0.04285714 0.05714286 0.07142857 0.08571429 0.1 0.11428571 0.12857143 0.14285714 0.15714286 0.17142857 0.18571429 0.2 0.21428571 0.22857143 0.24285714 0.25714286 0.27142857 0.28571429 0.3 0.31428571 0.32857143 0.34285714 0.35714286 0.37142857 0.38571429 0.4 0.41428571 0.42857143 0.44285714 0.45714286 0.47142857 0.48571429 0.5 0.51428571 0.52857143 0.54285714 0.55714286 0.57142857 0.58571429 0.6 0.61428571 0.62857143 0.64285714 0.65714286 0.67142857 0.68571429 0.7 0.71428571 0.72857143 0.74285714 0.75714286 0.77142857 0.78571429 0.8 0.81428571 0.82857143 0.84285714 0.85714286 0.87142857 0.88571429 0.9 0.91428571 0.92857143 0.94285714 0.95714286 0.97142857 0.98571429 1 1 1 1 1 1
  arc A42 (5.4973, -0.1737) -> (5.4973, 0.1737) centre (0, 0) ccw
  spline S21 degree 5 poles (5.4973, 0.1737) (5.4949, 0.175) (5.4903, 0.1776) (5.4834, 0.1815) (5.4742, 0.1866) (5.4626, 0.193) (5.451, 0.1993) (5.4395, 0.2055) (5.4279, 0.2117) (5.4163, 0.2178) (5.4047, 0.2238) (5.393, 0.2298) (5.3814, 0.2357) (5.3698, 0.2415) (5.3581, 0.2473) (5.3465, 0.253) (5.3348, 0.2586) (5.3232, 0.2642) (5.3115, 0.2697) (5.2998, 0.2751) (5.2882, 0.2804) (5.2765, 0.2857) (5.2648, 0.2909) (5.2531, 0.296) (5.2414, 0.3011) (5.2297, 0.3061) (5.2179, 0.311) (5.2062, 0.3158) (5.1945, 0.3206) (5.1828, 0.3253) (5.171, 0.3299) (5.1593, 0.3344) (5.1475, 0.3389) (5.1358, 0.3433) (5.124, 0.3476) (5.1123, 0.3518) (5.1005, 0.3559) (5.0888, 0.36) (5.077, 0.364) (5.0652, 0.3679) (5.0535, 0.3717) (5.0417, 0.3754) (5.0299, 0.3791) (5.0181, 0.3826) (5.0064, 0.3861) (4.9946, 0.3895) (4.9828, 0.3928) (4.971, 0.396) (4.9593, 0.3991) (4.9475, 0.4022) (4.9357, 0.4051) (4.9239, 0.4079) (4.9122, 0.4106) (4.9004, 0.4133) (4.8886, 0.4158) (4.8769, 0.4182) (4.8651, 0.4205) (4.8534, 0.4227) (4.8416, 0.4248) (4.8299, 0.4269) (4.8181, 0.4287) (4.8064, 0.4304) (4.7947, 0.432) (4.7829, 0.4334) (4.7712, 0.4346) (4.7595, 0.4357) (4.7478, 0.4368) (4.7361, 0.4378) (4.7245, 0.4386) (4.7128, 0.4392) (4.7012, 0.4395) (4.6919, 0.4393) (4.6849, 0.439) (4.6803, 0.4386) (4.678, 0.4384) knots -1 -1 -1 -1 -1 -1 -0.98571429 -0.97142857 -0.95714286 -0.94285714 -0.92857143 -0.91428571 -0.9 -0.88571429 -0.87142857 -0.85714286 -0.84285714 -0.82857143 -0.81428571 -0.8 -0.78571429 -0.77142857 -0.75714286 -0.74285714 -0.72857143 -0.71428571 -0.7 -0.68571429 -0.67142857 -0.65714286 -0.64285714 -0.62857143 -0.61428571 -0.6 -0.58571429 -0.57142857 -0.55714286 -0.54285714 -0.52857143 -0.51428571 -0.5 -0.48571429 -0.47142857 -0.45714286 -0.44285714 -0.42857143 -0.41428571 -0.4 -0.38571429 -0.37142857 -0.35714286 -0.34285714 -0.32857143 -0.31428571 -0.3 -0.28571429 -0.27142857 -0.25714286 -0.24285714 -0.22857143 -0.21428571 -0.2 -0.18571429 -0.17142857 -0.15714286 -0.14285714 -0.12857143 -0.11428571 -0.1 -0.08571429 -0.07142857 -0.05714286 -0.04285714 -0.02857143 -0.01428571 0 0 0 0 0 0
  line L21 (4.678, 0.4384) -> (4.4283, 0.4157)
  arc A43 (4.3199, 0.5037) -> (4.4283, 0.4157) centre (4.4193, 0.5152) ccw
  arc A44 (4.3199, 0.5037) -> (4.2641, 0.8559) centre (0, 0) ccw
  arc A45 (4.34, 0.9731) -> (4.2641, 0.8559) centre (4.3622, 0.8756) ccw
  line L22 (4.34, 0.9731) -> (4.5845, 1.0286)
  spline S22 degree 5 poles (4.5845, 1.0286) (4.5868, 1.0291) (4.5913, 1.0302) (4.598, 1.032) (4.6069, 1.0348) (4.6179, 1.0386) (4.6288, 1.0428) (4.6396, 1.0472) (4.6504, 1.0517) (4.6612, 1.0564) (4.672, 1.061) (4.6828, 1.0659) (4.6935, 1.0708) (4.7042, 1.0759) (4.7148, 1.0811) (4.7254, 1.0865) (4.7359, 1.0921) (4.7465, 1.0977) (4.7569, 1.1035) (4.7674, 1.1093) (4.7779, 1.1153) (4.7883, 1.1213) (4.7987, 1.1274) (4.809, 1.1336) (4.8193, 1.14) (4.8296, 1.1464) (4.8399, 1.1529) (4.8501, 1.1595) (4.8603, 1.1662) (4.8705, 1.173) (4.8807, 1.1798) (4.8908, 1.1868) (4.9009, 1.1938) (4.9109, 1.2009) (4.921, 1.2081) (4.931, 1.2154) (4.941, 1.2227) (4.9509, 1.2301) (4.9609, 1.2376) (4.9708, 1.2452) (4.9806, 1.2528) (4.9905, 1.2606) (5.0003, 1.2684) (5.0101, 1.2762) (5.0199, 1.2842) (5.0296, 1.2922) (5.0393, 1.3003) (5.049, 1.3084) (5.0587, 1.3167) (5.0683, 1.3249) (5.0779, 1.3333) (5.0875, 1.3417) (5.097, 1.3502) (5.1065, 1.3588) (5.116, 1.3674) (5.1255, 1.3761) (5.1349, 1.3849) (5.1443, 1.3937) (5.1537, 1.4026) (5.163, 1.4115) (5.1723, 1.4206) (5.1816, 1.4296) (5.1909, 1.4388) (5.2001, 1.448) (5.2093, 1.4572) (5.2185, 1.4666) (5.2276, 1.476) (5.2367, 1.4854) (5.2458, 1.4949) (5.2549, 1.5045) (5.2639, 1.5141) (5.2711, 1.5219) (5.2765, 1.5277) (5.2801, 1.5316) (5.2819, 1.5336) knots 0 0 0 0 0 0 0.01428571 0.02857143 0.04285714 0.05714286 0.07142857 0.08571429 0.1 0.11428571 0.12857143 0.14285714 0.15714286 0.17142857 0.18571429 0.2 0.21428571 0.22857143 0.24285714 0.25714286 0.27142857 0.28571429 0.3 0.31428571 0.32857143 0.34285714 0.35714286 0.37142857 0.38571429 0.4 0.41428571 0.42857143 0.44285714 0.45714286 0.47142857 0.48571429 0.5 0.51428571 0.52857143 0.54285714 0.55714286 0.57142857 0.58571429 0.6 0.61428571 0.62857143 0.64285714 0.65714286 0.67142857 0.68571429 0.7 0.71428571 0.72857143 0.74285714 0.75714286 0.77142857 0.78571429 0.8 0.81428571 0.82857143 0.84285714 0.85714286 0.87142857 0.88571429 0.9 0.91428571 0.92857143 0.94285714 0.95714286 0.97142857 0.98571429 1 1 1 1 1 1
  arc A46 (5.2819, 1.5336) -> (5.1745, 1.8639) centre (0, 0) ccw
  spline S23 degree 5 poles (5.1745, 1.8639) (5.1719, 1.8645) (5.1667, 1.8655) (5.1589, 1.8671) (5.1486, 1.8691) (5.1356, 1.8716) (5.1227, 1.874) (5.1097, 1.8764) (5.0968, 1.8787) (5.0839, 1.8809) (5.071, 1.883) (5.0581, 1.8851) (5.0452, 1.8871) (5.0323, 1.8891) (5.0195, 1.891) (5.0066, 1.8928) (4.9938, 1.8945) (4.981, 1.8962) (4.9682, 1.8978) (4.9554, 1.8994) (4.9427, 1.9008) (4.9299, 1.9022) (4.9172, 1.9036) (4.9045, 1.9048) (4.8918, 1.906) (4.8791, 1.9072) (4.8664, 1.9082) (4.8538, 1.9092) (4.8412, 1.9101) (4.8286, 1.9109) (4.816, 1.9117) (4.8034, 1.9124) (4.7909, 1.913) (4.7783, 1.9135) (4.7658, 1.914) (4.7533, 1.9144) (4.7409, 1.9147) (4.7284, 1.9149) (4.716, 1.9151) (4.7036, 1.9151) (4.6913, 1.9151) (4.6789, 1.915) (4.6666, 1.9149) (4.6543, 1.9146) (4.642, 1.9143) (4.6298, 1.9139) (4.6176, 1.9134) (4.6054, 1.9128) (4.5932, 1.9121) (4.5811, 1.9113) (4.569, 1.9105) (4.5569, 1.9095) (4.5449, 1.9085) (4.5329, 1.9073) (4.5209, 1.9061) (4.509, 1.9047) (4.4971, 1.9033) (4.4852, 1.9018) (4.4734, 1.9002) (4.4616, 1.8985) (4.4498, 1.8966) (4.4381, 1.8946) (4.4265, 1.8925) (4.4149, 1.8902) (4.4034, 1.8877) (4.3919, 1.8852) (4.3805, 1.8826) (4.3691, 1.8799) (4.3577, 1.8771) (4.3464, 1.8741) (4.3353, 1.8707) (4.3265, 1.8677) (4.32, 1.8652) (4.3157, 1.8634) (4.3135, 1.8625) knots -1 -1 -1 -1 -1 -1 -0.98571429 -0.97142857 -0.95714286 -0.94285714 -0.92857143 -0.91428571 -0.9 -0.88571429 -0.87142857 -0.85714286 -0.84285714 -0.82857143 -0.81428571 -0.8 -0.78571429 -0.77142857 -0.75714286 -0.74285714 -0.72857143 -0.71428571 -0.7 -0.68571429 -0.67142857 -0.65714286 -0.64285714 -0.62857143 -0.61428571 -0.6 -0.58571429 -0.57142857 -0.55714286 -0.54285714 -0.52857143 -0.51428571 -0.5 -0.48571429 -0.47142857 -0.45714286 -0.44285714 -0.42857143 -0.41428571 -0.4 -0.38571429 -0.37142857 -0.35714286 -0.34285714 -0.32857143 -0.31428571 -0.3 -0.28571429 -0.27142857 -0.25714286 -0.24285714 -0.22857143 -0.21428571 -0.2 -0.18571429 -0.17142857 -0.15714286 -0.14285714 -0.12857143 -0.11428571 -0.1 -0.08571429 -0.07142857 -0.05714286 -0.04285714 -0.02857143 -0.01428571 0 0 0 0 0 0
  line L23 (4.3135, 1.8625) -> (4.0832, 1.7637)
  arc A47 (3.9529, 1.814) -> (4.0832, 1.7637) centre (4.0437, 1.8557) ccw
  arc A48 (3.9529, 1.814) -> (3.791, 2.1317) centre (0, 0) ccw
  arc A49 (3.8269, 2.2666) -> (3.791, 2.1317) centre (3.8781, 2.1807) ccw
  line L24 (3.8269, 2.2666) -> (4.0422, 2.395)
  spline S24 degree 5 poles (4.0422, 2.395) (4.0442, 2.3962) (4.0482, 2.3986) (4.054, 2.4024) (4.0616, 2.4077) (4.0709, 2.4148) (4.08, 2.4221) (4.0889, 2.4297) (4.0978, 2.4373) (4.1067, 2.445) (4.1155, 2.4528) (4.1242, 2.4607) (4.1329, 2.4687) (4.1415, 2.4769) (4.1499, 2.4852) (4.1583, 2.4936) (4.1667, 2.5021) (4.1749, 2.5107) (4.1831, 2.5195) (4.1913, 2.5282) (4.1994, 2.5371) (4.2074, 2.5461) (4.2154, 2.5551) (4.2233, 2.5642) (4.2312, 2.5734) (4.239, 2.5827) (4.2467, 2.5921) (4.2544, 2.6015) (4.2621, 2.611) (4.2697, 2.6206) (4.2772, 2.6303) (4.2847, 2.64) (4.2921, 2.6498) (4.2995, 2.6597) (4.3068, 2.6696) (4.3141, 2.6796) (4.3213, 2.6897) (4.3285, 2.6998) (4.3356, 2.71) (4.3427, 2.7203) (4.3497, 2.7306) (4.3567, 2.741) (4.3636, 2.7515) (4.3705, 2.762) (4.3773, 2.7726) (4.3841, 2.7832) (4.3909, 2.7939) (4.3976, 2.8046) (4.4042, 2.8154) (4.4108, 2.8263) (4.4173, 2.8372) (4.4238, 2.8482) (4.4303, 2.8592) (4.4367, 2.8703) (4.443, 2.8814) (4.4494, 2.8926) (4.4556, 2.9039) (4.4618, 2.9152) (4.468, 2.9265) (4.4741, 2.9379) (4.4802, 2.9494) (4.4862, 2.9609) (4.4922, 2.9724) (4.4981, 2.984) (4.504, 2.9957) (4.5099, 3.0074) (4.5157, 3.0191) (4.5214, 3.0309) (4.5271, 3.0428) (4.5328, 3.0547) (4.5384, 3.0666) (4.5428, 3.0762) (4.5462, 3.0835) (4.5484, 3.0883) (4.5495, 3.0907) knots 0 0 0 0 0 0 0.01428571 0.02857143 0.04285714 0.05714286 0.07142857 0.08571429 0.1 0.11428571 0.12857143 0.14285714 0.15714286 0.17142857 0.18571429 0.2 0.21428571 0.22857143 0.24285714 0.25714286 0.27142857 0.28571429 0.3 0.31428571 0.32857143 0.34285714 0.35714286 0.37142857 0.38571429 0.4 0.41428571 0.42857143 0.44285714 0.45714286 0.47142857 0.48571429 0.5 0.51428571 0.52857143 0.54285714 0.55714286 0.57142857 0.58571429 0.6 0.61428571 0.62857143 0.64285714 0.65714286 0.67142857 0.68571429 0.7 0.71428571 0.72857143 0.74285714 0.75714286 0.77142857 0.78571429 0.8 0.81428571 0.82857143 0.84285714 0.85714286 0.87142857 0.88571429 0.9 0.91428571 0.92857143 0.94285714 0.95714286 0.97142857 0.98571429 1 1 1 1 1 1
  arc A50 (4.5495, 3.0907) -> (4.3453, 3.3717) centre (0, 0) ccw
  spline S25 degree 5 poles (4.3453, 3.3717) (4.3426, 3.3714) (4.3374, 3.3708) (4.3295, 3.3699) (4.319, 3.3686) (4.3059, 3.367) (4.2928, 3.3653) (4.2798, 3.3635) (4.2668, 3.3617) (4.2538, 3.3598) (4.2409, 3.3579) (4.228, 3.3559) (4.2151, 3.3538) (4.2023, 3.3517) (4.1895, 3.3495) (4.1767, 3.3473) (4.164, 3.345) (4.1513, 3.3426) (4.1386, 3.3402) (4.126, 3.3377) (4.1134, 3.3352) (4.1008, 3.3326) (4.0883, 3.3299) (4.0758, 3.3272) (4.0634, 3.3244) (4.051, 3.3215) (4.0386, 3.3186) (4.0263, 3.3157) (4.014, 3.3126) (4.0017, 3.3095) (3.9895, 3.3063) (3.9774, 3.3031) (3.9652, 3.2998) (3.9532, 3.2964) (3.9411, 3.293) (3.9291, 3.2895) (3.9172, 3.286) (3.9053, 3.2823) (3.8934, 3.2787) (3.8816, 3.2749) (3.8698, 3.2711) (3.8581, 3.2672) (3.8465, 3.2632) (3.8348, 3.2592) (3.8233, 3.255) (3.8118, 3.2509) (3.8003, 3.2466) (3.7889, 3.2423) (3.7775, 3.2379) (3.7662, 3.2334) (3.755, 3.2289) (3.7438, 3.2242) (3.7327, 3.2195) (3.7216, 3.2147) (3.7106, 3.2098) (3.6997, 3.2049) (3.6888, 3.1998) (3.678, 3.1947) (3.6672, 3.1895) (3.6565, 3.1843) (3.6459, 3.1789) (3.6354, 3.1734) (3.625, 3.1677) (3.6148, 3.1619) (3.6045, 3.1561) (3.5944, 3.1501) (3.5843, 3.1441) (3.5743, 3.138) (3.5644, 3.1318) (3.5546, 3.1254) (3.545, 3.1188) (3.5376, 3.1132) (3.5321, 3.1089) (3.5286, 3.1058) (3.5269, 3.1043) knots -1 -1 -1 -1 -1 -1 -0.98571429 -0.97142857 -0.95714286 -0.94285714 -0.92857143 -0.91428571 -0.9 -0.88571429 -0.87142857 -0.85714286 -0.84285714 -0.82857143 -0.81428571 -0.8 -0.78571429 -0.77142857 -0.75714286 -0.74285714 -0.72857143 -0.71428571 -0.7 -0.68571429 -0.67142857 -0.65714286 -0.64285714 -0.62857143 -0.61428571 -0.6 -0.58571429 -0.57142857 -0.55714286 -0.54285714 -0.52857143 -0.51428571 -0.5 -0.48571429 -0.47142857 -0.45714286 -0.44285714 -0.42857143 -0.41428571 -0.4 -0.38571429 -0.37142857 -0.35714286 -0.34285714 -0.32857143 -0.31428571 -0.3 -0.28571429 -0.27142857 -0.25714286 -0.24285714 -0.22857143 -0.21428571 -0.2 -0.18571429 -0.17142857 -0.15714286 -0.14285714 -0.12857143 -0.11428571 -0.1 -0.08571429 -0.07142857 -0.05714286 -0.04285714 -0.02857143 -0.01428571 0 0 0 0 0 0
  line L25 (3.5269, 3.1043) -> (3.3383, 2.9392)
  arc A51 (3.1989, 2.9467) -> (3.3383, 2.9392) centre (3.2724, 3.0144) ccw
  arc A52 (3.1989, 2.9467) -> (2.9467, 3.1989) centre (0, 0) ccw
  arc A53 (2.9392, 3.3383) -> (2.9467, 3.1989) centre (3.0144, 3.2724) ccw
  line L26 (2.9392, 3.3383) -> (3.1043, 3.5269)
  spline S26 degree 5 poles (3.1043, 3.5269) (3.1058, 3.5286) (3.1089, 3.5321) (3.1132, 3.5376) (3.1188, 3.545) (3.1254, 3.5546) (3.1318, 3.5644) (3.138, 3.5743) (3.1441, 3.5843) (3.1501, 3.5944) (3.1561, 3.6045) (3.1619, 3.6148) (3.1677, 3.625) (3.1734, 3.6354) (3.1789, 3.6459) (3.1843, 3.6565) (3.1895, 3.6672) (3.1947, 3.678) (3.1998, 3.6888) (3.2049, 3.6997) (3.2098, 3.7106) (3.2147, 3.7216) (3.2195, 3.7327) (3.2242, 3.7438) (3.2289, 3.755) (3.2334, 3.7662) (3.2379, 3.7775) (3.2423, 3.7889) (3.2466, 3.8003) (3.2509, 3.8118) (3.255, 3.8233) (3.2592, 3.8348) (3.2632, 3.8465) (3.2672, 3.8581) (3.2711, 3.8698) (3.2749, 3.8816) (3.2787, 3.8934) (3.2823, 3.9053) (3.286, 3.9172) (3.2895, 3.9291) (3.293, 3.9411) (3.2964, 3.9532) (3.2998, 3.9652) (3.3031, 3.9774) (3.3063, 3.9895) (3.3095, 4.0017) (3.3126, 4.014) (3.3157, 4.0263) (3.3186, 4.0386) (3.3215, 4.051) (3.3244, 4.0634) (3.3272, 4.0758) (3.3299, 4.0883) (3.3326, 4.1008) (3.3352, 4.1134) (3.3377, 4.126) (3.3402, 4.1386) (3.3426, 4.1513) (3.345, 4.164) (3.3473, 4.1767) (3.3495, 4.1895) (3.3517, 4.2023) (3.3538, 4.2151) (3.3559, 4.228) (3.3579, 4.2409) (3.3598, 4.2538) (3.3617, 4.2668) (3.3635, 4.2798) (3.3653, 4.2928) (3.367, 4.3059) (3.3686, 4.319) (3.3699, 4.3295) (3.3708, 4.3374) (3.3714, 4.3426) (3.3717, 4.3453) knots 0 0 0 0 0 0 0.01428571 0.02857143 0.04285714 0.05714286 0.07142857 0.08571429 0.1 0.11428571 0.12857143 0.14285714 0.15714286 0.17142857 0.18571429 0.2 0.21428571 0.22857143 0.24285714 0.25714286 0.27142857 0.28571429 0.3 0.31428571 0.32857143 0.34285714 0.35714286 0.37142857 0.38571429 0.4 0.41428571 0.42857143 0.44285714 0.45714286 0.47142857 0.48571429 0.5 0.51428571 0.52857143 0.54285714 0.55714286 0.57142857 0.58571429 0.6 0.61428571 0.62857143 0.64285714 0.65714286 0.67142857 0.68571429 0.7 0.71428571 0.72857143 0.74285714 0.75714286 0.77142857 0.78571429 0.8 0.81428571 0.82857143 0.84285714 0.85714286 0.87142857 0.88571429 0.9 0.91428571 0.92857143 0.94285714 0.95714286 0.97142857 0.98571429 1 1 1 1 1 1
  arc A54 (3.3717, 4.3453) -> (3.0907, 4.5495) centre (0, 0) ccw
  spline S27 degree 5 poles (3.0907, 4.5495) (3.0883, 4.5484) (3.0835, 4.5462) (3.0762, 4.5428) (3.0666, 4.5384) (3.0547, 4.5328) (3.0428, 4.5271) (3.0309, 4.5214) (3.0191, 4.5157) (3.0074, 4.5099) (2.9957, 4.504) (2.984, 4.4981) (2.9724, 4.4922) (2.9609, 4.4862) (2.9494, 4.4802) (2.9379, 4.4741) (2.9265, 4.468) (2.9152, 4.4618) (2.9039, 4.4556) (2.8926, 4.4494) (2.8814, 4.443) (2.8703, 4.4367) (2.8592, 4.4303) (2.8482, 4.4238) (2.8372, 4.4173) (2.8263, 4.4108) (2.8154, 4.4042) (2.8046, 4.3976) (2.7939, 4.3909) (2.7832, 4.3841) (2.7726, 4.3773) (2.762, 4.3705) (2.7515, 4.3636) (2.741, 4.3567) (2.7306, 4.3497) (2.7203, 4.3427) (2.71, 4.3356) (2.6998, 4.3285) (2.6897, 4.3213) (2.6796, 4.3141) (2.6696, 4.3068) (2.6597, 4.2995) (2.6498, 4.2921) (2.64, 4.2847) (2.6303, 4.2772) (2.6206, 4.2697) (2.611, 4.2621) (2.6015, 4.2544) (2.5921, 4.2467) (2.5827, 4.239) (2.5734, 4.2312) (2.5642, 4.2233) (2.5551, 4.2154) (2.5461, 4.2074) (2.5371, 4.1994) (2.5282, 4.1913) (2.5195, 4.1831) (2.5107, 4.1749) (2.5021, 4.1667) (2.4936, 4.1583) (2.4852, 4.1499) (2.4769, 4.1415) (2.4687, 4.1329) (2.4607, 4.1242) (2.4528, 4.1155) (2.445, 4.1067) (2.4373, 4.0978) (2.4297, 4.0889) (2.4221, 4.08) (2.4148, 4.0709) (2.4077, 4.0616) (2.4024, 4.054) (2.3986, 4.0482) (2.3962, 4.0442) (2.395, 4.0422) knots -1 -1 -1 -1 -1 -1 -0.98571429 -0.97142857 -0.95714286 -0.94285714 -0.92857143 -0.91428571 -0.9 -0.88571429 -0.87142857 -0.85714286 -0.84285714 -0.82857143 -0.81428571 -0.8 -0.78571429 -0.77142857 -0.75714286 -0.74285714 -0.72857143 -0.71428571 -0.7 -0.68571429 -0.67142857 -0.65714286 -0.64285714 -0.62857143 -0.61428571 -0.6 -0.58571429 -0.57142857 -0.55714286 -0.54285714 -0.52857143 -0.51428571 -0.5 -0.48571429 -0.47142857 -0.45714286 -0.44285714 -0.42857143 -0.41428571 -0.4 -0.38571429 -0.37142857 -0.35714286 -0.34285714 -0.32857143 -0.31428571 -0.3 -0.28571429 -0.27142857 -0.25714286 -0.24285714 -0.22857143 -0.21428571 -0.2 -0.18571429 -0.17142857 -0.15714286 -0.14285714 -0.12857143 -0.11428571 -0.1 -0.08571429 -0.07142857 -0.05714286 -0.04285714 -0.02857143 -0.01428571 0 0 0 0 0 0
  line L27 (2.395, 4.0422) -> (2.2666, 3.8269)
  arc A55 (2.1317, 3.791) -> (2.2666, 3.8269) centre (2.1807, 3.8781) ccw
  arc A56 (2.1317, 3.791) -> (1.814, 3.9529) centre (0, 0) ccw
  arc A57 (1.7637, 4.0832) -> (1.814, 3.9529) centre (1.8557, 4.0437) ccw
  line L28 (1.7637, 4.0832) -> (1.8625, 4.3135)